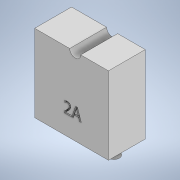
# Autodesk Inventor part: Support_2A
Saved by Autodesk Inventor 2021 (Build 250183000, 183)
## iProperties
Created: 2021-04-14
Part Number: Support_2A
Material: Generic
Document SubType Name: Modeling
Designer: Jawal
Density: 1 g/cm^3
Appearance: Default
Author: Jawal
Autodesk Inventor part; units mm, degrees
note: some values were not read from the file. Chosen so that the rebuilt part matches the saved one: direction of "Emboss1".
ref_plane "YZ Plane" through (0, 0, 0) normal (1, 0, 0) x (0, 1, 0)
ref_plane "XZ Plane" through (0, 0, 0) normal (0, 1, 0) x (-1, 0, 0)
ref_plane "XY Plane" through (0, 0, 0) normal (0, 0, 1) x (1, 0, 0)
sketch "Sketch1" plane through (0, 0, 0) normal (1, 0, 0) x (0, 1, 0)
  line L0 (11.4385, 5) -> (-11.4385, 5)
  line L1 (-11.4385, 5) -> (-11.4385, -5)
  line L2 (-11.4385, -5) -> (11.4385, -5)
  line L3 (11.4385, -5) -> (11.4385, 5)
  point P0 (0, 0)
  dimension "d0" = 22.877
  dimension "d1" = 11.4385
  dimension "d3" = 10
  dimension "d4" = 5
  constraints: 8 end point, 2 parallel, 1 horizontal, 1 perpendicular
  measures "d0" distance of L1.end L2.end
  measures "d1" distance from line of point (0, 0) L3
  measures "d3" distance of L2.end L0.start
  measures "d4" distance from line of point (0, 0) L0
extrude "Extrusion1" add sketch "Sketch1" along normal blind 20
sketch "Sketch2" plane through (0, -11.4385, -5) normal (0, -1, 0) x (1, 0, 0)
  circle A0 centre (16.5, 5) radius 1.5
  line L0 (20, 10) -> (20, 0) projected
  point P0 (0, 5)
  dimension "d7" = 3
  dimension "d8" = 3.5
  constraints: 1 centre point
  measures "d7" diameter of A0
  measures "d8" distance from line of L0 A0.centre
extrude "Extrusion2" add sketch "Sketch2" along normal blind 3
sketch "Sketch4" plane through (0, -11.4385, 5) normal (0, 0, 1) x (1, 0, 0)
  line L0 (7.8092, 8.2906) -> (13.0725, 8.2906) construction
  line L1 (13.0725, 8.2906) -> (13.0725, 3.3647) construction
  line L2 (13.0725, 3.3647) -> (7.8092, 3.3647) construction
  line L3 (7.8092, 3.3647) -> (7.8092, 8.2906) construction
  line L4 (9.9112, 5.1784) -> (8.0315, 5.1784)
  line L5 (8.0315, 5.1784) -> (8.0315, 5.6107)
  spline S0 degree 2 poles (8.0315, 5.6107) (8.234, 5.8008) (8.5947, 6.1541) (8.7676, 6.3443) knots 0 0 0 1 2 2 2
  spline S1 degree 2 poles (8.7676, 6.3443) (9.1158, 6.7271) (9.3702, 7.1865) (9.3702, 7.4311) knots 0 0 0 1 2 2 2
  spline S2 degree 2 poles (9.3702, 7.4311) (9.3702, 7.5595) (9.2912, 7.7522) (9.2196, 7.8139) knots 0 0 0 1 2 2 2
  spline S3 degree 2 poles (9.2196, 7.8139) (9.1479, 7.8757) (8.9602, 7.9374) (8.8466, 7.9374) knots 0 0 0 1 2 2 2
  spline S4 degree 2 poles (8.8466, 7.9374) (8.7379, 7.9374) (8.5156, 7.8831) (8.4143, 7.8411) knots 0 0 0 1 2 2 2
  spline S5 degree 2 poles (8.4143, 7.8411) (8.3279, 7.8065) (8.1673, 7.7077) (8.1179, 7.6731) knots 0 0 0 1 2 2 2
  line L6 (8.1179, 7.6731) -> (8.0957, 7.6731)
  line L7 (8.0957, 7.6731) -> (8.0957, 8.1078)
  spline S6 degree 2 poles (8.0957, 8.1078) (8.2217, 8.1696) (8.6737, 8.2906) (8.8762, 8.2906) knots 0 0 0 1 2 2 2
  spline S7 degree 2 poles (8.8762, 8.2906) (9.3036, 8.2906) (9.7852, 7.8386) (9.7852, 7.4533) knots 0 0 0 1 2 2 2
  spline S8 degree 2 poles (9.7852, 7.4533) (9.7852, 7.273) (9.7012, 6.9716) (9.6271, 6.8432) knots 0 0 0 1 2 2 2
  spline S9 degree 2 poles (9.6271, 6.8432) (9.553, 6.7098) (9.3381, 6.448) (9.2196, 6.322) knots 0 0 0 1 2 2 2
  spline S10 degree 2 poles (9.2196, 6.322) (9.0269, 6.1121) (8.5551, 5.6625) (8.4143, 5.5316) knots 0 0 0 1 2 2 2
  line L8 (8.4143, 5.5316) -> (9.9112, 5.5316)
  line L9 (9.9112, 5.5316) -> (9.9112, 5.1784)
  line L10 (10.0767, 5.1784) -> (11.1042, 8.2264)
  line L11 (11.1042, 8.2264) -> (11.6031, 8.2264)
  line L12 (11.6031, 8.2264) -> (12.6307, 5.1784)
  line L13 (12.6307, 5.1784) -> (12.2033, 5.1784)
  line L14 (12.2033, 5.1784) -> (11.9267, 6.0306)
  line L15 (11.9267, 6.0306) -> (10.7633, 6.0306)
  line L16 (10.7633, 6.0306) -> (10.4867, 5.1784)
  line L17 (10.4867, 5.1784) -> (10.0767, 5.1784)
  line L18 (11.8156, 6.3764) -> (11.3438, 7.8114)
  line L19 (11.3438, 7.8114) -> (10.8745, 6.3764)
  line L20 (10.8745, 6.3764) -> (11.8156, 6.3764)
  point P0 (0, 11.4385)
  constraints: 2 other
emboss "Emboss1" sketch "Sketch4" operation cut depth 1 direction (0, 0, -1)
sketch "Sketch5" plane through (0, 11.4385, 5) normal (0, 1, 0) x (1, 0, 0)
  line L0 (20, 0) -> (20, 10) projected
  line L1 (0, 0) -> (20, 0) projected
  line L2 (20, 10) -> (0, 10)
  line L3 (0, 10) -> (0, 0)
  line L4 (0, 0) -> (20, 0)
  line L5 (20, 0) -> (20, 10)
  point P0 (0, 5)
  constraints: 8 end point, 2 parallel, 1 horizontal, 1 perpendicular
extrude "Extrusion4" cut sketch "Sketch5" against normal blind 1.877
sketch "Sketch6" plane through (0, -11.4385, 5) normal (0, 0, 1) x (1, 0, 0)
  line L0 (20, 21) -> (0, 21) projected
  circle A0 centre (11, 21) radius 1.5
  line L1 (20, 21) -> (20, 0) projected
  point P0 (0, 11.4385)
  point P1 (9.5, 21)
  point P2 (12.5, 21)
  dimension "d20" = 3
  dimension "d21" = 9
  constraints: 1 centre point, 1 point on line
  measures "d20" diameter of A0
  measures "d21" distance from line of L1 A0.centre
extrude "Extrusion5" cut sketch "Sketch6" against normal up to surface (10 mm away) contours A0 L0 picked at (11.2986, 20.4689)
equation "\"d1\" = 0.5 * d0"
equation "\"d4\" = 0.5 * d3"
body "Solid1"
